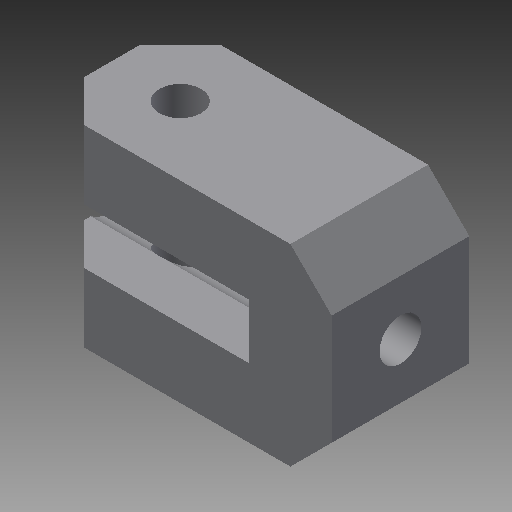
# Autodesk Inventor part: cross head
Saved by Autodesk Inventor 2017 SP1 (Build 210196100, 196)
## iProperties
Created: 2017-06-14
Part Number: cross head
Material: Generic
Document SubType Name: Modeling
Designer: RMcComber
Density: 1 g/cm^3
Appearance: Default
Author: RMcComber
Autodesk Inventor part; units mm, degrees
ref_plane "YZ Plane" through (0, 0, 0) normal (1, 0, 0) x (0, 1, 0)
ref_plane "XZ Plane" through (0, 0, 0) normal (0, 1, 0) x (-1, 0, 0)
ref_plane "XY Plane" through (0, 0, 0) normal (0, 0, 1) x (1, 0, 0)
sketch "Sketch1" plane through (0, 0, 0) normal (0, 0, 1) x (1, 0, 0)
  line L0 (0, 0) -> (-30, 0)
  line L1 (-30, 0) -> (-30, 10)
  line L2 (-30, 10) -> (0, 10)
  line L3 (0, 10) -> (0, 0)
  line L4 (0, 10) -> (12, 10)
  line L5 (12, 10) -> (12, -18)
  line L6 (12, -18) -> (0, -18)
  line L7 (0, -18) -> (0, 10)
  line L8 (0, -18) -> (-30, -18)
  line L9 (-30, -18) -> (-30, -8)
  line L10 (-30, -8) -> (0, -8)
  line L11 (0, -8) -> (0, -18)
  dimension "d0" = 8
  dimension "d1" = 10
  dimension "d2" = 10
  dimension "d3" = 12
  dimension "d4" = 30
  constraints: 24 end point, 7 parallel, 3 horizontal, 3 perpendicular
  measures "d0" distance between parallel lines of L10 L0
  measures "d1" distance of L0.end L1.end
  measures "d2" distance of L8.end L9.end
  measures "d3" distance between parallel lines of L7 L5
  measures "d4" distance of L1.end L2.end
extrude "Extrusion1" add sketch "Sketch1" along normal blind 20
sketch "Sketch2" plane through (0, -8, 0) normal (-1, 0, 0) x (0, 0, 1)
  line L0 (20, 8) -> (20, 0) projected
  line L1 (0, 8) -> (0, 0) projected
  line L2 (0, 4) -> (20, 4) construction
  circle A0 centre (10, 4) radius 3.05
  dimension "d7" = 6.1
  constraints: 3 midpoint, 2 end point, 1 centre point
  measures "d7" diameter of A0
extrude "Extrusion2" cut sketch "Sketch2" against normal through all
sketch "Sketch3" plane through (-30, 10, 0) normal (0, 1, 0) x (1, 0, 0)
  line L0 (30, 0) -> (30, -20) projected
  line L1 (30, -10) -> (10, -10) construction
  circle A0 centre (10, -10) radius 3.05
  circle A1 centre (10, -10) radius 8.5 construction
  line L2 (42, 0) -> (42, -20) projected
  dimension "d10" = 17
  dimension "d11" = 6.1
  dimension "d12" = 20
  dimension "d24" = 11.5
  dimension "d25" = 32
  constraints: 2 centre point, 2 coincident, 2 end point, 1 midpoint, 1 perpendicular
  measures "d10" diameter of A1
  measures "d11" diameter of A0
  measures "d12" distance of L1.start L1.end
  measures "d24" distance edge to line of A1 L0
  measures "d25" distance from line of L2 A0.centre
extrude "Extrusion3" cut sketch "Sketch3" against normal through all
sketch "Sketch4" plane through (-30, 0, 0) normal (-1, 0, 0) x (0, 0, 1)
  circle A0 centre (10, -4) radius 3.05 projected
  circle A1 centre (10, -4) radius 5
  dimension "d15" = 10
  constraints: 1 centre point, 1 coincident
  measures "d15" diameter of A1
extrude "Extrusion4" cut sketch "Sketch4" against normal up to surface (30 mm away)
chamfer "Chamfer1" distance 6 angle 45 4 edges at (-30, 5, 0) (-30, 5, 20) (-30, -13, 0) (-30, -13, 20)
chamfer "Chamfer2" distance 6 angle 45 2 edges at (12, 10, 10) (12, -18, 10)
body "Solid1"
